Autodesk Fusion 360 part; units mm, degrees
(part 2 of 5)
sketch "Sketch2" plane through (0, 0, 22) normal (0, 0, 1) x (-1, 0, 0)
  line L0 (-259.9009, 59) -> (-249.9009, 59)
  line L1 (-249.9009, 59) -> (-249.9009, 53)
  line L2 (-249.9009, 53) -> (-259.9009, 53)
  line L3 (-259.9009, 53) -> (-259.9009, 59)
  arc A0 (-260.2748, 92.3293) -> (-257.2248, 89.2793) centre (-257.2248, 92.3293) ccw
  line L4 (-260.2748, 92.3293) -> (-260.2748, 97.7293)
  arc A1 (-257.2248, 100.7793) -> (-260.2748, 97.7293) centre (-257.2248, 97.7293) ccw
  line L5 (-257.2248, 100.7793) -> (-251.8248, 100.7793)
  arc A2 (-248.7748, 97.7293) -> (-251.8248, 100.7793) centre (-251.8248, 97.7293) ccw
  line L6 (-248.7748, 97.7293) -> (-248.7748, 92.3293)
  arc A3 (-251.8248, 89.2793) -> (-248.7748, 92.3293) centre (-251.8248, 92.3293) ccw
  line L7 (-251.8248, 89.2793) -> (-257.2248, 89.2793)
  line L8 (-263.1698, 97.5713) -> (-263.1698, 92.1713)
  arc A4 (-266.2198, 89.1213) -> (-263.1698, 92.1713) centre (-266.2198, 92.1713) ccw
  line L9 (-266.2198, 89.1213) -> (-271.6198, 89.1213)
  arc A5 (-274.6698, 92.1713) -> (-271.6198, 89.1213) centre (-271.6198, 92.1713) ccw
  line L10 (-274.6698, 92.1713) -> (-274.6698, 97.5713)
  arc A6 (-271.6198, 100.6213) -> (-274.6698, 97.5713) centre (-271.6198, 97.5713) ccw
  line L11 (-271.6198, 100.6213) -> (-266.2198, 100.6213)
  arc A7 (-263.1698, 97.5713) -> (-266.2198, 100.6213) centre (-266.2198, 97.5713) ccw
  circle A8 centre (-270.3911, 55.7056) radius 3
  circle A9 centre (-281.5411, 55.7956) radius 3
  line L12 (-248.7148, 86.5518) -> (-247.9448, 86.5518)
  arc A10 (-247.6948, 86.5414) -> (-247.9448, 86.5518) centre (-247.9448, 83.5518) ccw
  arc A11 (-247.4448, 86.5518) -> (-247.6948, 86.5414) centre (-247.4448, 83.5518) ccw
  line L13 (-247.4448, 86.5518) -> (-246.6748, 86.5518)
  arc A12 (-246.4248, 86.5414) -> (-246.6748, 86.5518) centre (-246.6748, 83.5518) ccw
  arc A13 (-246.1748, 86.5518) -> (-246.4248, 86.5414) centre (-246.1748, 83.5518) ccw
  line L14 (-246.1748, 86.5518) -> (-245.4048, 86.5518)
  arc A14 (-245.1548, 86.5414) -> (-245.4048, 86.5518) centre (-245.4048, 83.5518) ccw
  arc A15 (-244.9048, 86.5518) -> (-245.1548, 86.5414) centre (-244.9048, 83.5518) ccw
  line L15 (-244.9048, 86.5518) -> (-244.1348, 86.5518)
  arc A16 (-243.8848, 86.5414) -> (-244.1348, 86.5518) centre (-244.1348, 83.5518) ccw
  arc A17 (-243.6348, 86.5518) -> (-243.8848, 86.5414) centre (-243.6348, 83.5518) ccw
  line L16 (-243.6348, 86.5518) -> (-242.8648, 86.5518)
  arc A18 (-242.6148, 86.5414) -> (-242.8648, 86.5518) centre (-242.8648, 83.5518) ccw
  arc A19 (-242.3648, 86.5518) -> (-242.6148, 86.5414) centre (-242.3648, 83.5518) ccw
  line L17 (-242.3648, 86.5518) -> (-241.5148, 86.5518)
  arc A20 (-241.3048, 86.5445) -> (-241.5148, 86.5518) centre (-241.5148, 83.5518) ccw
  arc A21 (-241.0948, 86.5518) -> (-241.3048, 86.5445) centre (-241.0948, 83.5518) ccw
  line L18 (-241.0948, 86.5518) -> (-240.3248, 86.5518)
  arc A22 (-240.0748, 86.5414) -> (-240.3248, 86.5518) centre (-240.3248, 83.5518) ccw
  arc A23 (-239.8248, 86.5518) -> (-240.0748, 86.5414) centre (-239.8248, 83.5518) ccw
  line L19 (-239.8248, 86.5518) -> (-239.0548, 86.5518)
  arc A24 (-238.8048, 86.5414) -> (-239.0548, 86.5518) centre (-239.0548, 83.5518) ccw
  arc A25 (-238.5548, 86.5518) -> (-238.8048, 86.5414) centre (-238.5548, 83.5518) ccw
  line L20 (-238.5548, 86.5518) -> (-237.7848, 86.5518)
  arc A26 (-237.5348, 86.5414) -> (-237.7848, 86.5518) centre (-237.7848, 83.5518) ccw
  arc A27 (-237.2848, 86.5518) -> (-237.5348, 86.5414) centre (-237.2848, 83.5518) ccw
  line L21 (-237.2848, 86.5518) -> (-236.5148, 86.5518)
  arc A28 (-236.2648, 86.5414) -> (-236.5148, 86.5518) centre (-236.5148, 83.5518) ccw
  arc A29 (-236.0148, 86.5518) -> (-236.2648, 86.5414) centre (-236.0148, 83.5518) ccw
  line L22 (-236.0148, 86.5518) -> (-235.2448, 86.5518)
  arc A30 (-234.9948, 86.5414) -> (-235.2448, 86.5518) centre (-235.2448, 83.5518) ccw
  arc A31 (-234.7448, 86.5518) -> (-234.9948, 86.5414) centre (-234.7448, 83.5518) ccw
  line L23 (-234.7448, 86.5518) -> (-233.9748, 86.5518)
  arc A32 (-233.7248, 86.5414) -> (-233.9748, 86.5518) centre (-233.9748, 83.5518) ccw
  arc A33 (-233.4748, 86.5518) -> (-233.7248, 86.5414) centre (-233.4748, 83.5518) ccw
  line L24 (-233.4748, 86.5518) -> (-232.7048, 86.5518)
  arc A34 (-232.4548, 86.5414) -> (-232.7048, 86.5518) centre (-232.7048, 83.5518) ccw
  arc A35 (-232.2048, 86.5518) -> (-232.4548, 86.5414) centre (-232.2048, 83.5518) ccw
  line L25 (-232.2048, 86.5518) -> (-199.377, 86.5518)
  line L26 (-199.377, 86.5518) -> (-199.377, 118.6521)
  line L27 (-199.377, 118.6521) -> (-338.527, 118.6521)
  line L28 (-338.527, 118.6521) -> (-338.527, 36.7921)
  line L29 (-338.527, 36.7921) -> (-199.377, 36.7921)
  line L30 (-199.377, 36.7921) -> (-199.377, 62.5518)
  line L31 (-199.377, 62.5518) -> (-232.2048, 62.5518)
  arc A36 (-232.4548, 62.5622) -> (-232.2048, 62.5518) centre (-232.2048, 65.5518) ccw
  arc A37 (-232.7048, 62.5518) -> (-232.4548, 62.5622) centre (-232.7048, 65.5518) ccw
  line L32 (-232.7048, 62.5518) -> (-233.4748, 62.5518)
  arc A38 (-233.633, 62.556) -> (-233.4748, 62.5518) centre (-233.4748, 65.5518) ccw
  line L33 (-233.633, 62.556) -> (-233.633, 53)
  line L34 (-233.633, 53) -> (-245.633, 53)
  line L35 (-245.633, 53) -> (-245.633, 62.5518)
  line L36 (-245.633, 62.5518) -> (-246.1748, 62.5518)
  arc A39 (-246.4248, 62.5622) -> (-246.1748, 62.5518) centre (-246.1748, 65.5518) ccw
  arc A40 (-246.6748, 62.5518) -> (-246.4248, 62.5622) centre (-246.6748, 65.5518) ccw
  line L37 (-246.6748, 62.5518) -> (-247.4448, 62.5518)
  arc A41 (-247.6948, 62.5622) -> (-247.4448, 62.5518) centre (-247.4448, 65.5518) ccw
  arc A42 (-247.9448, 62.5518) -> (-247.6948, 62.5622) centre (-247.9448, 65.5518) ccw
  line L38 (-247.9448, 62.5518) -> (-248.7148, 62.5518)
  arc A43 (-248.9648, 62.5622) -> (-248.7148, 62.5518) centre (-248.7148, 65.5518) ccw
  arc A44 (-249.2148, 62.5518) -> (-248.9648, 62.5622) centre (-249.2148, 65.5518) ccw
  line L39 (-249.2148, 62.5518) -> (-252.4198, 62.5518)
  arc A45 (-253.4198, 63.5518) -> (-252.4198, 62.5518) centre (-252.4198, 63.5518) ccw
  line L40 (-253.4198, 63.5518) -> (-253.4198, 68.5418)
  arc A46 (-253.4094, 68.7918) -> (-253.4198, 68.5418) centre (-250.4198, 68.5418) ccw
  arc A47 (-253.4198, 69.0418) -> (-253.4094, 68.7918) centre (-250.4198, 69.0418) ccw
  line L41 (-253.4198, 69.0418) -> (-253.4198, 69.8118)
  arc A48 (-253.4094, 70.0618) -> (-253.4198, 69.8118) centre (-250.4198, 69.8118) ccw
  arc A49 (-253.4198, 70.3118) -> (-253.4094, 70.0618) centre (-250.4198, 70.3118) ccw
  line L42 (-253.4198, 70.3118) -> (-253.4198, 71.0818)
  arc A50 (-253.4094, 71.3318) -> (-253.4198, 71.0818) centre (-250.4198, 71.0818) ccw
  arc A51 (-253.4198, 71.5818) -> (-253.4094, 71.3318) centre (-250.4198, 71.5818) ccw
  line L43 (-253.4198, 71.5818) -> (-253.4198, 72.3518)
  arc A52 (-253.4094, 72.6018) -> (-253.4198, 72.3518) centre (-250.4198, 72.3518) ccw
  arc A53 (-253.4198, 72.8518) -> (-253.4094, 72.6018) centre (-250.4198, 72.8518) ccw
  line L44 (-253.4198, 72.8518) -> (-253.4198, 73.6218)
  arc A54 (-253.4094, 73.8718) -> (-253.4198, 73.6218) centre (-250.4198, 73.6218) ccw
  arc A55 (-253.4198, 74.1218) -> (-253.4094, 73.8718) centre (-250.4198, 74.1218) ccw
  line L45 (-253.4198, 74.1218) -> (-253.4198, 74.8918)
  arc A56 (-253.4094, 75.1418) -> (-253.4198, 74.8918) centre (-250.4198, 74.8918) ccw
  arc A57 (-253.4198, 75.3918) -> (-253.4094, 75.1418) centre (-250.4198, 75.3918) ccw
  line L46 (-253.4198, 75.3918) -> (-253.4198, 76.1618)
  arc A58 (-253.4094, 76.4118) -> (-253.4198, 76.1618) centre (-250.4198, 76.1618) ccw
  arc A59 (-253.4198, 76.6618) -> (-253.4094, 76.4118) centre (-250.4198, 76.6618) ccw
  line L47 (-253.4198, 76.6618) -> (-253.4198, 77.4318)
  arc A60 (-253.4094, 77.6818) -> (-253.4198, 77.4318) centre (-250.4198, 77.4318) ccw
  arc A61 (-253.4198, 77.9318) -> (-253.4094, 77.6818) centre (-250.4198, 77.9318) ccw
  line L48 (-253.4198, 77.9318) -> (-253.4198, 78.7018)
  arc A62 (-253.4094, 78.9518) -> (-253.4198, 78.7018) centre (-250.4198, 78.7018) ccw
  arc A63 (-253.4198, 79.2018) -> (-253.4094, 78.9518) centre (-250.4198, 79.2018) ccw
  line L49 (-253.4198, 79.2018) -> (-253.4198, 79.9718)
  arc A64 (-253.4094, 80.2218) -> (-253.4198, 79.9718) centre (-250.4198, 79.9718) ccw
  arc A65 (-253.4198, 80.4718) -> (-253.4094, 80.2218) centre (-250.4198, 80.4718) ccw
  line L50 (-253.4198, 80.4718) -> (-253.4198, 85.5518)
  arc A66 (-252.4198, 86.5518) -> (-253.4198, 85.5518) centre (-252.4198, 85.5518) ccw
  line L51 (-252.4198, 86.5518) -> (-249.2148, 86.5518)
  arc A67 (-248.9648, 86.5414) -> (-249.2148, 86.5518) centre (-249.2148, 83.5518) ccw
  arc A68 (-248.7148, 86.5518) -> (-248.9648, 86.5414) centre (-248.7148, 83.5518) ccw
  line L52 (-266.6857, 52.6914) -> (-273.6857, 52.6914) construction
  line L53 (-273.6857, 52.6914) -> (-273.6857, 49.6914) construction
  line L54 (-273.6857, 49.6914) -> (-266.6857, 49.6914) construction
  line L55 (-266.6857, 49.6914) -> (-266.6857, 52.6914) construction
  line L56 (-266.6857, 52.6914) -> (-273.6857, 52.6914) construction
  line L57 (-273.6857, 52.6914) -> (-273.6857, 49.6914) construction
  line L58 (-273.6857, 49.6914) -> (-266.6857, 49.6914) construction
  line L59 (-266.6857, 49.6914) -> (-266.6857, 52.6914) construction
  line L60 (-277.8686, 52.3387) -> (-283.3242, 52.3387) construction
  line L61 (-283.3242, 52.3387) -> (-283.3242, 49.9371) construction
  line L62 (-283.3242, 49.9371) -> (-277.8686, 49.9371) construction
  line L63 (-277.8686, 49.9371) -> (-277.8686, 52.3387) construction
  line L64 (-251.7291, 106.4343) -> (-265.6571, 106.4343) construction
  line L65 (-265.6571, 106.4343) -> (-265.6571, 101.6182) construction
  line L66 (-265.6571, 101.6182) -> (-251.7291, 101.6182) construction
  line L67 (-251.7291, 101.6182) -> (-251.7291, 106.4343) construction
  line L68 (-265.6571, 106.1257) -> (-277.7028, 106.1257) construction
  line L69 (-277.7028, 106.1257) -> (-277.7028, 101.6182) construction
  line L70 (-277.7028, 101.6182) -> (-265.6571, 101.6182) construction
  line L71 (-265.6571, 101.6182) -> (-265.6571, 106.1257) construction
  dimension "d91" = 2
  dimension "d93" = 2
  dimension "d95" = 2
  dimension "d97" = 2
  dimension "d99" = 2
  text T0 "Status" font "Arial" height 2 align left top in box 7 x 3 at (-266.6857, 52.6914) x (-1, 0) y (0, -1) spacing 1
  text T1 "Power" font "Arial" height 2 align left top in box 5.4557 x 2.4015 at (-277.8686, 52.3387) x (-1, 0) y (0, -1) spacing 1
  text T2 "Boot" font "Arial" height 2 align left top in box 13.928 x 4.8161 at (-251.7291, 106.4343) x (-1, 0) y (0, -1) spacing 1
  text T3 "Reset" font "Arial" height 2 align left top in box 12.0457 x 4.5075 at (-265.6571, 106.1257) x (-1, 0) y (0, -1) spacing 1
extrude "Extrude2" cut sketch "Sketch2" against normal blind 0.5 text T0 T1 T2 T3
sketch "Sketch3" plane through (0, 0, 22) normal (0, 0, 1) x (-1, 0, 0)
  line L0 (-248.7148, 86.5518) -> (-247.9448, 86.5518)
  arc A0 (-247.6948, 86.5414) -> (-247.9448, 86.5518) centre (-247.9448, 83.5518) ccw
  arc A1 (-247.4448, 86.5518) -> (-247.6948, 86.5414) centre (-247.4448, 83.5518) ccw
  line L1 (-247.4448, 86.5518) -> (-246.6748, 86.5518)
  arc A2 (-246.4248, 86.5414) -> (-246.6748, 86.5518) centre (-246.6748, 83.5518) ccw
  arc A3 (-246.1748, 86.5518) -> (-246.4248, 86.5414) centre (-246.1748, 83.5518) ccw
  line L2 (-246.1748, 86.5518) -> (-245.4048, 86.5518)
  arc A4 (-245.1548, 86.5414) -> (-245.4048, 86.5518) centre (-245.4048, 83.5518) ccw
  arc A5 (-244.9048, 86.5518) -> (-245.1548, 86.5414) centre (-244.9048, 83.5518) ccw
  line L3 (-244.9048, 86.5518) -> (-244.1348, 86.5518)
  arc A6 (-243.8848, 86.5414) -> (-244.1348, 86.5518) centre (-244.1348, 83.5518) ccw
  arc A7 (-243.6348, 86.5518) -> (-243.8848, 86.5414) centre (-243.6348, 83.5518) ccw
  line L4 (-243.6348, 86.5518) -> (-242.8648, 86.5518)
  arc A8 (-242.6148, 86.5414) -> (-242.8648, 86.5518) centre (-242.8648, 83.5518) ccw
  arc A9 (-242.3648, 86.5518) -> (-242.6148, 86.5414) centre (-242.3648, 83.5518) ccw
  line L5 (-242.3648, 86.5518) -> (-241.5148, 86.5518)
  arc A10 (-241.3048, 86.5445) -> (-241.5148, 86.5518) centre (-241.5148, 83.5518) ccw
  arc A11 (-241.0948, 86.5518) -> (-241.3048, 86.5445) centre (-241.0948, 83.5518) ccw
  line L6 (-241.0948, 86.5518) -> (-240.3248, 86.5518)
  arc A12 (-240.0748, 86.5414) -> (-240.3248, 86.5518) centre (-240.3248, 83.5518) ccw
  arc A13 (-239.8248, 86.5518) -> (-240.0748, 86.5414) centre (-239.8248, 83.5518) ccw
  line L7 (-239.8248, 86.5518) -> (-239.0548, 86.5518)
  arc A14 (-238.8048, 86.5414) -> (-239.0548, 86.5518) centre (-239.0548, 83.5518) ccw
  arc A15 (-238.5548, 86.5518) -> (-238.8048, 86.5414) centre (-238.5548, 83.5518) ccw
  line L8 (-238.5548, 86.5518) -> (-237.7848, 86.5518)
  arc A16 (-237.5348, 86.5414) -> (-237.7848, 86.5518) centre (-237.7848, 83.5518) ccw
  arc A17 (-237.2848, 86.5518) -> (-237.5348, 86.5414) centre (-237.2848, 83.5518) ccw
  line L9 (-237.2848, 86.5518) -> (-236.5148, 86.5518)
  arc A18 (-236.2648, 86.5414) -> (-236.5148, 86.5518) centre (-236.5148, 83.5518) ccw
  arc A19 (-236.0148, 86.5518) -> (-236.2648, 86.5414) centre (-236.0148, 83.5518) ccw
  line L10 (-236.0148, 86.5518) -> (-235.2448, 86.5518)
  arc A20 (-234.9948, 86.5414) -> (-235.2448, 86.5518) centre (-235.2448, 83.5518) ccw
  arc A21 (-234.7448, 86.5518) -> (-234.9948, 86.5414) centre (-234.7448, 83.5518) ccw
  line L11 (-234.7448, 86.5518) -> (-233.9748, 86.5518)
  arc A22 (-233.7248, 86.5414) -> (-233.9748, 86.5518) centre (-233.9748, 83.5518) ccw
  arc A23 (-233.4748, 86.5518) -> (-233.7248, 86.5414) centre (-233.4748, 83.5518) ccw
  line L12 (-233.4748, 86.5518) -> (-232.7048, 86.5518)
  arc A24 (-232.4548, 86.5414) -> (-232.7048, 86.5518) centre (-232.7048, 83.5518) ccw
  arc A25 (-232.2048, 86.5518) -> (-232.4548, 86.5414) centre (-232.2048, 83.5518) ccw
  line L13 (-232.2048, 86.5518) -> (-199.377, 86.5518)
  line L14 (-199.377, 86.5518) -> (-199.377, 118.6521)
  line L15 (-199.377, 118.6521) -> (-338.527, 118.6521)
  line L16 (-338.527, 118.6521) -> (-338.527, 36.7921)
  line L17 (-338.527, 36.7921) -> (-199.377, 36.7921)
  line L18 (-199.377, 36.7921) -> (-199.377, 62.5518)
  line L19 (-199.377, 62.5518) -> (-232.2048, 62.5518)
  arc A26 (-232.4548, 62.5622) -> (-232.2048, 62.5518) centre (-232.2048, 65.5518) ccw
  arc A27 (-232.7048, 62.5518) -> (-232.4548, 62.5622) centre (-232.7048, 65.5518) ccw
  line L20 (-232.7048, 62.5518) -> (-233.4748, 62.5518)
  arc A28 (-233.633, 62.556) -> (-233.4748, 62.5518) centre (-233.4748, 65.5518) ccw
  line L21 (-233.633, 62.556) -> (-233.633, 53)
  line L22 (-233.633, 53) -> (-245.633, 53)
  line L23 (-245.633, 53) -> (-245.633, 62.5518)
  line L24 (-245.633, 62.5518) -> (-246.1748, 62.5518)
  arc A29 (-246.4248, 62.5622) -> (-246.1748, 62.5518) centre (-246.1748, 65.5518) ccw
  arc A30 (-246.6748, 62.5518) -> (-246.4248, 62.5622) centre (-246.6748, 65.5518) ccw
  line L25 (-246.6748, 62.5518) -> (-247.4448, 62.5518)
  arc A31 (-247.6948, 62.5622) -> (-247.4448, 62.5518) centre (-247.4448, 65.5518) ccw
  arc A32 (-247.9448, 62.5518) -> (-247.6948, 62.5622) centre (-247.9448, 65.5518) ccw
  line L26 (-247.9448, 62.5518) -> (-248.7148, 62.5518)
  arc A33 (-248.9648, 62.5622) -> (-248.7148, 62.5518) centre (-248.7148, 65.5518) ccw
  arc A34 (-249.2148, 62.5518) -> (-248.9648, 62.5622) centre (-249.2148, 65.5518) ccw
  line L27 (-249.2148, 62.5518) -> (-252.4198, 62.5518)
  arc A35 (-253.4198, 63.5518) -> (-252.4198, 62.5518) centre (-252.4198, 63.5518) ccw
  line L28 (-253.4198, 63.5518) -> (-253.4198, 68.5418)
  arc A36 (-253.4094, 68.7918) -> (-253.4198, 68.5418) centre (-250.4198, 68.5418) ccw
  arc A37 (-253.4198, 69.0418) -> (-253.4094, 68.7918) centre (-250.4198, 69.0418) ccw
  line L29 (-253.4198, 69.0418) -> (-253.4198, 69.8118)
  arc A38 (-253.4094, 70.0618) -> (-253.4198, 69.8118) centre (-250.4198, 69.8118) ccw
  arc A39 (-253.4198, 70.3118) -> (-253.4094, 70.0618) centre (-250.4198, 70.3118) ccw
  line L30 (-253.4198, 70.3118) -> (-253.4198, 71.0818)
  arc A40 (-253.4094, 71.3318) -> (-253.4198, 71.0818) centre (-250.4198, 71.0818) ccw
  arc A41 (-253.4198, 71.5818) -> (-253.4094, 71.3318) centre (-250.4198, 71.5818) ccw
  line L31 (-253.4198, 71.5818) -> (-253.4198, 72.3518)
  arc A42 (-253.4094, 72.6018) -> (-253.4198, 72.3518) centre (-250.4198, 72.3518) ccw
  arc A43 (-253.4198, 72.8518) -> (-253.4094, 72.6018) centre (-250.4198, 72.8518) ccw
  line L32 (-253.4198, 72.8518) -> (-253.4198, 73.6218)
  arc A44 (-253.4094, 73.8718) -> (-253.4198, 73.6218) centre (-250.4198, 73.6218) ccw
  arc A45 (-253.4198, 74.1218) -> (-253.4094, 73.8718) centre (-250.4198, 74.1218) ccw
  line L33 (-253.4198, 74.1218) -> (-253.4198, 74.8918)
  arc A46 (-253.4094, 75.1418) -> (-253.4198, 74.8918) centre (-250.4198, 74.8918) ccw
  arc A47 (-253.4198, 75.3918) -> (-253.4094, 75.1418) centre (-250.4198, 75.3918) ccw
  line L34 (-253.4198, 75.3918) -> (-253.4198, 76.1618)
  arc A48 (-253.4094, 76.4118) -> (-253.4198, 76.1618) centre (-250.4198, 76.1618) ccw
  arc A49 (-253.4198, 76.6618) -> (-253.4094, 76.4118) centre (-250.4198, 76.6618) ccw
  line L35 (-253.4198, 76.6618) -> (-253.4198, 77.4318)
  arc A50 (-253.4094, 77.6818) -> (-253.4198, 77.4318) centre (-250.4198, 77.4318) ccw
  arc A51 (-253.4198, 77.9318) -> (-253.4094, 77.6818) centre (-250.4198, 77.9318) ccw
  line L36 (-253.4198, 77.9318) -> (-253.4198, 78.7018)
  arc A52 (-253.4094, 78.9518) -> (-253.4198, 78.7018) centre (-250.4198, 78.7018) ccw
  arc A53 (-253.4198, 79.2018) -> (-253.4094, 78.9518) centre (-250.4198, 79.2018) ccw
  line L37 (-253.4198, 79.2018) -> (-253.4198, 79.9718)
  arc A54 (-253.4094, 80.2218) -> (-253.4198, 79.9718) centre (-250.4198, 79.9718) ccw
  arc A55 (-253.4198, 80.4718) -> (-253.4094, 80.2218) centre (-250.4198, 80.4718) ccw
  line L38 (-253.4198, 80.4718) -> (-253.4198, 85.5518)
  arc A56 (-252.4198, 86.5518) -> (-253.4198, 85.5518) centre (-252.4198, 85.5518) ccw
  line L39 (-252.4198, 86.5518) -> (-249.2148, 86.5518)
  arc A57 (-248.9648, 86.5414) -> (-249.2148, 86.5518) centre (-249.2148, 83.5518) ccw
  arc A58 (-248.7148, 86.5518) -> (-248.9648, 86.5414) centre (-248.7148, 83.5518) ccw
  circle A59 centre (-281.5411, 55.7956) radius 3
  circle A60 centre (-270.3911, 55.7056) radius 3
  line L40 (-263.1698, 97.5713) -> (-263.1698, 92.1713)
  arc A61 (-266.2198, 89.1213) -> (-263.1698, 92.1713) centre (-266.2198, 92.1713) ccw
  line L41 (-266.2198, 89.1213) -> (-271.6198, 89.1213)
  arc A62 (-274.6698, 92.1713) -> (-271.6198, 89.1213) centre (-271.6198, 92.1713) ccw
  line L42 (-274.6698, 92.1713) -> (-274.6698, 97.5713)
  arc A63 (-271.6198, 100.6213) -> (-274.6698, 97.5713) centre (-271.6198, 97.5713) ccw
  line L43 (-271.6198, 100.6213) -> (-266.2198, 100.6213)
  arc A64 (-263.1698, 97.5713) -> (-266.2198, 100.6213) centre (-266.2198, 97.5713) ccw
  arc A65 (-260.2748, 92.3293) -> (-257.2248, 89.2793) centre (-257.2248, 92.3293) ccw
  line L44 (-260.2748, 92.3293) -> (-260.2748, 97.7293)
  arc A66 (-257.2248, 100.7793) -> (-260.2748, 97.7293) centre (-257.2248, 97.7293) ccw
  line L45 (-257.2248, 100.7793) -> (-251.8248, 100.7793)
  arc A67 (-248.7748, 97.7293) -> (-251.8248, 100.7793) centre (-251.8248, 97.7293) ccw
  line L46 (-248.7748, 97.7293) -> (-248.7748, 92.3293)
  arc A68 (-251.8248, 89.2793) -> (-248.7748, 92.3293) centre (-251.8248, 92.3293) ccw
  line L47 (-251.8248, 89.2793) -> (-257.2248, 89.2793)
  line L48 (-259.9009, 59) -> (-249.9009, 59)
  line L49 (-249.9009, 59) -> (-249.9009, 53)
  line L50 (-249.9009, 53) -> (-259.9009, 53)
  line L51 (-259.9009, 53) -> (-259.9009, 59)
  line L52 (-265.9218, 103.6182) -> (-265.6571, 103.6182)
  line L53 (-265.6571, 103.6182) -> (-265.6571, 101.6182)
  spline S0 degree 3 poles (-266.9504, 101.6721) (-266.9947, 101.6939) (-267.085, 101.7384) (-267.1432, 101.8206) (-267.1728, 101.8624) knots 0 0 0 0 0.014568 0.029686 0.029686 0.029686 0.029686
  spline S1 degree 3 poles (-267.1728, 101.8624) (-267.1971, 101.9093) (-267.246, 102.004) (-267.2527, 102.1103) (-267.256, 102.1639) knots 0 0 0 0 0.015657 0.031584 0.031584 0.031584 0.031584
  spline S2 degree 3 poles (-272.5725, 103.4081) (-272.5883, 103.4076) (-272.6244, 103.4063) (-272.6602, 103.4014) (-272.6803, 103.3986) knots 0 0 0 0 0.004747 0.010826 0.010826 0.010826 0.010826
  line L54 (-272.6803, 103.3986) -> (-272.7158, 103.6155)
  spline S3 degree 3 poles (-271.4306, 103.3781) (-271.4615, 103.349) (-271.529, 103.2853) (-271.5634, 103.1987) (-271.5821, 103.1517) knots 0 0 0 0 0.012573 0.027537 0.027537 0.027537 0.027537
  line L55 (-271.5821, 103.1517) -> (-271.8358, 103.183)
  spline S4 degree 3 poles (-271.8358, 103.183) (-271.8125, 103.2523) (-271.7674, 103.3862) (-271.6636, 103.4819) (-271.6134, 103.5282) knots 0 0 0 0 0.021523 0.041652 0.041652 0.041652 0.041652
  spline S5 degree 3 poles (-254.1602, 103.651) (-254.0648, 103.644) (-253.88, 103.6304) (-253.7373, 103.5128) (-253.6684, 103.4559) knots 0 0 0 0 0.027936 0.054087 0.054087 0.054087 0.054087
  spline S6 degree 3 poles (-253.6684, 103.4559) (-253.6138, 103.3793) (-253.4945, 103.2119) (-253.4856, 103.0056) (-253.4808, 102.8938) knots 0 0 0 0 0.027653 0.060391 0.060391 0.060391 0.060391
  spline S7 degree 3 poles (-253.4808, 102.8938) (-253.4864, 102.7719) (-253.4967, 102.5476) (-253.6394, 102.3759) (-253.7045, 102.2976) knots 0 0 0 0 0.035471 0.065242 0.065242 0.065242 0.065242
  spline S8 degree 3 poles (-253.7045, 102.2976) (-253.7713, 102.2507) (-253.9079, 102.1545) (-254.0748, 102.1427) (-254.1602, 102.1367) knots 0 0 0 0 0.023996 0.049149 0.049149 0.049149 0.049149
  spline S9 degree 3 poles (-254.1602, 102.1367) (-254.2544, 102.1439) (-254.438, 102.1581) (-254.5796, 102.2753) (-254.6486, 102.3324) knots 0 0 0 0 0.027586 0.05378 0.05378 0.05378 0.05378
  spline S10 degree 3 poles (-254.6486, 102.3324) (-254.7038, 102.4073) (-254.8221, 102.5675) (-254.8326, 102.767) (-254.8382, 102.8734) knots 0 0 0 0 0.027308 0.058452 0.058452 0.058452 0.058452
  spline S11 degree 3 poles (-254.8382, 102.8734) (-254.8366, 102.9577) (-254.8336, 103.1095) (-254.7787, 103.2506) (-254.7543, 103.3133) knots 0 0 0 0 0.025071 0.045099 0.045099 0.045099 0.045099
  spline S12 degree 3 poles (-254.7543, 103.3133) (-254.7231, 103.3638) (-254.6604, 103.4652) (-254.5603, 103.5298) (-254.5101, 103.5623) knots 0 0 0 0 0.017574 0.035265 0.035265 0.035265 0.035265
  spline S13 degree 3 poles (-254.5101, 103.5623) (-254.4552, 103.5882) (-254.3443, 103.6404) (-254.2219, 103.6474) (-254.1602, 103.651) knots 0 0 0 0 0.018034 0.036399 0.036399 0.036399 0.036399
  spline S14 degree 3 poles (-255.7141, 103.651) (-255.6186, 103.644) (-255.4339, 103.6304) (-255.2912, 103.5128) (-255.2223, 103.4559) knots 0 0 0 0 0.027936 0.054087 0.054087 0.054087 0.054087
  spline S15 degree 3 poles (-255.2223, 103.4559) (-255.1677, 103.3793) (-255.0484, 103.2119) (-255.0395, 103.0056) (-255.0347, 102.8938) knots 0 0 0 0 0.027653 0.060391 0.060391 0.060391 0.060391
  spline S16 degree 3 poles (-255.0347, 102.8938) (-255.0403, 102.7719) (-255.0506, 102.5476) (-255.1933, 102.3759) (-255.2584, 102.2976) knots 0 0 0 0 0.035471 0.065242 0.065242 0.065242 0.065242
  spline S17 degree 3 poles (-255.2584, 102.2976) (-255.3251, 102.2507) (-255.4618, 102.1545) (-255.6287, 102.1427) (-255.7141, 102.1367) knots 0 0 0 0 0.023996 0.049149 0.049149 0.049149 0.049149
  spline S18 degree 3 poles (-255.7141, 102.1367) (-255.8083, 102.1439) (-255.9918, 102.1581) (-256.1335, 102.2753) (-256.2025, 102.3324) knots 0 0 0 0 0.027586 0.05378 0.05378 0.05378 0.05378
  spline S19 degree 3 poles (-256.2025, 102.3324) (-256.2577, 102.4073) (-256.376, 102.5675) (-256.3865, 102.767) (-256.3921, 102.8734) knots 0 0 0 0 0.027308 0.058452 0.058452 0.058452 0.058452
  spline S20 degree 3 poles (-256.3921, 102.8734) (-256.3905, 102.9577) (-256.3875, 103.1095) (-256.3326, 103.2506) (-256.3082, 103.3133) knots 0 0 0 0 0.025071 0.045099 0.045099 0.045099 0.045099
  spline S21 degree 3 poles (-256.3082, 103.3133) (-256.277, 103.3638) (-256.2143, 103.4652) (-256.1142, 103.5298) (-256.064, 103.5623) knots 0 0 0 0 0.017574 0.035265 0.035265 0.035265 0.035265
  spline S22 degree 3 poles (-256.064, 103.5623) (-256.0091, 103.5882) (-255.8982, 103.6404) (-255.7758, 103.6474) (-255.7141, 103.651) knots 0 0 0 0 0.018034 0.036399 0.036399 0.036399 0.036399
  spline S23 degree 3 poles (-280.2888, 51.9699) (-280.1933, 51.9629) (-280.0086, 51.9493) (-279.8659, 51.8317) (-279.797, 51.7748) knots 0 0 0 0 0.027936 0.054087 0.054087 0.054087 0.054087
  spline S24 degree 3 poles (-279.797, 51.7748) (-279.7424, 51.6982) (-279.6231, 51.5308) (-279.6142, 51.3245) (-279.6094, 51.2127) knots 0 0 0 0 0.027653 0.060391 0.060391 0.060391 0.060391
  spline S25 degree 3 poles (-279.6094, 51.2127) (-279.615, 51.0908) (-279.6253, 50.8665) (-279.768, 50.6949) (-279.8331, 50.6165) knots 0 0 0 0 0.035471 0.065242 0.065242 0.065242 0.065242
  spline S26 degree 3 poles (-279.8331, 50.6165) (-279.8998, 50.5696) (-280.0365, 50.4734) (-280.2034, 50.4616) (-280.2888, 50.4556) knots 0 0 0 0 0.023996 0.049149 0.049149 0.049149 0.049149
  spline S27 degree 3 poles (-280.2888, 50.4556) (-280.383, 50.4628) (-280.5665, 50.477) (-280.7082, 50.5942) (-280.7772, 50.6513) knots 0 0 0 0 0.027586 0.05378 0.05378 0.05378 0.05378
  spline S28 degree 3 poles (-280.7772, 50.6513) (-280.8324, 50.7262) (-280.9507, 50.8864) (-280.9612, 51.0859) (-280.9668, 51.1923) knots 0 0 0 0 0.027308 0.058452 0.058452 0.058452 0.058452
  spline S29 degree 3 poles (-280.9668, 51.1923) (-280.9652, 51.2766) (-280.9622, 51.4284) (-280.9073, 51.5696) (-280.8829, 51.6322) knots 0 0 0 0 0.025071 0.045099 0.045099 0.045099 0.045099
  spline S30 degree 3 poles (-280.8829, 51.6322) (-280.8517, 51.6827) (-280.789, 51.7841) (-280.6889, 51.8488) (-280.6387, 51.8812) knots 0 0 0 0 0.017574 0.035265 0.035265 0.035265 0.035265
  spline S31 degree 3 poles (-280.6387, 51.8812) (-280.5838, 51.9071) (-280.4729, 51.9593) (-280.3505, 51.9663) (-280.2888, 51.9699) knots 0 0 0 0 0.018034 0.036399 0.036399 0.036399 0.036399
  line L56 (-282.0719, 50.8225) -> (-281.7785, 51.9371)
  line L57 (-281.7785, 51.9371) -> (-281.5221, 51.9371)
  line L58 (-281.5221, 51.9371) -> (-281.0787, 50.4883)
  line L59 (-281.0787, 50.4883) -> (-281.3324, 50.4883)
  line L60 (-281.3324, 50.4883) -> (-281.563, 51.3246)
  line L61 (-281.563, 51.3246) -> (-281.6489, 51.6356)
  spline S32 degree 3 poles (-281.6489, 51.6356) (-281.6561, 51.6069) (-281.6809, 51.5072) (-281.7061, 51.4077) (-281.724, 51.3369) knots 0 0 0 0 0.008892 0.030805 0.030805 0.030805 0.030805
  line L62 (-281.724, 51.3369) -> (-281.9545, 50.4883)
  line L63 (-281.9545, 50.4883) -> (-282.2069, 50.4883)
  line L64 (-282.2069, 50.4883) -> (-282.4238, 51.3287)
  line L65 (-282.4238, 51.3287) -> (-282.4961, 51.6056)
  line L66 (-282.4961, 51.6056) -> (-282.5794, 51.326)
  line L67 (-282.5794, 51.326) -> (-282.8277, 50.4883)
  line L68 (-282.8277, 50.4883) -> (-283.0664, 50.4883)
  line L69 (-283.0664, 50.4883) -> (-282.6135, 51.9371)
  line L70 (-282.6135, 51.9371) -> (-282.3584, 51.9371)
  line L71 (-282.3584, 51.9371) -> (-282.1278, 51.0695)
  line L72 (-282.1278, 51.0695) -> (-282.0719, 50.8225)
  spline S33 degree 3 poles (-266.5439, 101.6182) (-266.6229, 101.6188) (-266.7608, 101.6199) (-266.8937, 101.6565) (-266.9504, 101.6721) knots 0 0 0 0 0.023572 0.041164 0.041164 0.041164 0.041164
  spline S34 degree 3 poles (-266.7955, 51.4083) (-266.7649, 51.3532) (-266.7026, 51.2412) (-266.6914, 51.1136) (-266.6857, 51.0489) knots 0 0 0 0 0.018713 0.037965 0.037965 0.037965 0.037965
  line L73 (-266.6857, 51.0489) -> (-266.9354, 51.027)
  spline S35 degree 3 poles (-266.9354, 51.027) (-266.9424, 51.0735) (-266.9556, 51.1605) (-266.9981, 51.2375) (-267.0179, 51.2733) knots 0 0 0 0 0.013975 0.026155 0.026155 0.026155 0.026155
  spline S36 degree 3 poles (-267.0179, 51.2733) (-267.0438, 51.3044) (-267.0993, 51.3709) (-267.1775, 51.4087) (-267.2191, 51.4288) knots 0 0 0 0 0.012002 0.025694 0.025694 0.025694 0.025694
  spline S37 degree 3 poles (-267.2191, 51.4288) (-267.267, 51.4461) (-267.3661, 51.482) (-267.4715, 51.486) (-267.5261, 51.4881) knots 0 0 0 0 0.015163 0.031432 0.031432 0.031432 0.031432
  spline S38 degree 3 poles (-267.5261, 51.4881) (-267.574, 51.4867) (-267.6653, 51.4839) (-267.7522, 51.4563) (-267.7935, 51.4431) knots 0 0 0 0 0.014301 0.027232 0.027232 0.027232 0.027232
  spline S39 degree 3 poles (-267.7935, 51.4431) (-267.8289, 51.4277) (-267.8954, 51.3988) (-267.9436, 51.3448) (-267.9661, 51.3197) knots 0 0 0 0 0.011435 0.021444 0.021444 0.021444 0.021444
  spline S40 degree 3 poles (-267.9661, 51.3197) (-267.9826, 51.2931) (-268.0152, 51.2406) (-268.0202, 51.1789) (-268.0227, 51.1484) knots 0 0 0 0 0.009237 0.018267 0.018267 0.018267 0.018267
  spline S41 degree 3 poles (-268.0227, 51.1484) (-268.0206, 51.1183) (-268.0164, 51.0588) (-267.984, 51.0087) (-267.9681, 50.9841) knots 0 0 0 0 0.008921 0.017573 0.017573 0.017573 0.017573
  spline S42 degree 3 poles (-267.9681, 50.9841) (-267.9451, 50.9609) (-267.8935, 50.909) (-267.8256, 50.8814) (-267.788, 50.866) knots 0 0 0 0 0.009698 0.021725 0.021725 0.021725 0.021725
  spline S43 degree 3 poles (-267.788, 50.866) (-267.7451, 50.8523) (-267.6278, 50.8147) (-267.5079, 50.7864) (-267.432, 50.7685) knots 0 0 0 0 0.013533 0.036931 0.036931 0.036931 0.036931
  spline S44 degree 3 poles (-267.432, 50.7685) (-267.353, 50.7496) (-267.2209, 50.7181) (-267.0961, 50.665) (-267.0459, 50.6437) knots 0 0 0 0 0.024297 0.040637 0.040637 0.040637 0.040637
  spline S45 degree 3 poles (-267.0459, 50.6437) (-267.0019, 50.6183) (-266.9185, 50.5701) (-266.86, 50.4936) (-266.8324, 50.4575) knots 0 0 0 0 0.015064 0.02858 0.02858 0.02858 0.02858
  spline S46 degree 3 poles (-266.8324, 50.4575) (-266.8119, 50.419) (-266.7704, 50.3411) (-266.7649, 50.2531) (-266.7621, 50.2085) knots 0 0 0 0 0.012908 0.026139 0.026139 0.026139 0.026139
  spline S47 degree 3 poles (-266.7621, 50.2085) (-266.7658, 50.1586) (-266.7734, 50.0579) (-266.823, 49.9698) (-266.8481, 49.9254) knots 0 0 0 0 0.014805 0.02991 0.02991 0.02991 0.02991
  spline S48 degree 3 poles (-266.8481, 49.9254) (-266.8809, 49.8838) (-266.9489, 49.7977) (-267.0479, 49.7501) (-267.0991, 49.7255) knots 0 0 0 0 0.01568 0.032466 0.032466 0.032466 0.032466
  spline S49 degree 3 poles (-267.0991, 49.7255) (-267.1566, 49.7056) (-267.2755, 49.6646) (-267.4012, 49.6598) (-267.4661, 49.6573) knots 0 0 0 0 0.018164 0.037509 0.037509 0.037509 0.037509
  spline S50 degree 3 poles (-267.4661, 49.6573) (-267.5365, 49.6597) (-267.6709, 49.6642) (-267.7979, 49.7081) (-267.8583, 49.7289) knots 0 0 0 0 0.021001 0.040071 0.040071 0.040071 0.040071
  spline S51 degree 3 poles (-267.8583, 49.7289) (-267.9112, 49.755) (-268.0142, 49.8056) (-268.0851, 49.8958) (-268.1196, 49.9397) knots 0 0 0 0 0.017437 0.033952 0.033952 0.033952 0.033952
  spline S52 degree 3 poles (-268.1196, 49.9397) (-268.1465, 49.9881) (-268.2012, 50.0862) (-268.2122, 50.1981) (-268.2178, 50.2549) knots 0 0 0 0 0.016416 0.033327 0.033327 0.033327 0.033327
  line L74 (-268.2178, 50.2549) -> (-267.964, 50.274)
  spline S53 degree 3 poles (-267.964, 50.274) (-267.9545, 50.2158) (-267.9365, 50.1062) (-267.861, 50.0254) (-267.8256, 49.9875) knots 0 0 0 0 0.017238 0.032462 0.032462 0.032462 0.032462
  spline S54 degree 3 poles (-267.8256, 49.9875) (-267.778, 49.9593) (-267.6711, 49.896) (-267.5463, 49.8925) (-267.477, 49.8906) knots 0 0 0 0 0.016321 0.036707 0.036707 0.036707 0.036707
  spline S55 degree 3 poles (-267.477, 49.8906) (-267.4061, 49.8917) (-267.2818, 49.8936) (-267.1735, 49.9531) (-267.1271, 49.9786) knots 0 0 0 0 0.02087 0.036564 0.036564 0.036564 0.036564
  spline S56 degree 3 poles (-267.1271, 49.9786) (-267.095, 50.0086) (-267.0332, 50.0666) (-267.0224, 50.1504) (-267.0172, 50.1907) knots 0 0 0 0 0.012728 0.024562 0.024562 0.024562 0.024562
  spline S57 degree 3 poles (-267.0172, 50.1907) (-267.0204, 50.225) (-267.0265, 50.2928) (-267.0723, 50.3431) (-267.095, 50.3681) knots 0 0 0 0 0.010013 0.019843 0.019843 0.019843 0.019843
  spline S58 degree 3 poles (-267.095, 50.3681) (-267.1403, 50.3933) (-267.2648, 50.4627) (-267.4049, 50.492) (-267.494, 50.5107) knots 0 0 0 0 0.01549 0.042576 0.042576 0.042576 0.042576
  spline S59 degree 3 poles (-267.494, 50.5107) (-267.5854, 50.5311) (-267.7357, 50.5646) (-267.8801, 50.6175) (-267.9367, 50.6382) knots 0 0 0 0 0.028046 0.046113 0.046113 0.046113 0.046113
  spline S60 degree 3 poles (-267.9367, 50.6382) (-267.99, 50.6653) (-268.0899, 50.716) (-268.1613, 50.802) (-268.1946, 50.8422) knots 0 0 0 0 0.017708 0.033187 0.033187 0.033187 0.033187
  spline S61 degree 3 poles (-268.1946, 50.8422) (-268.2189, 50.8854) (-268.2684, 50.9738) (-268.2746, 51.075) (-268.2778, 51.1266) knots 0 0 0 0 0.014678 0.02998 0.02998 0.02998 0.02998
  spline S62 degree 3 poles (-268.2778, 51.1266) (-268.2738, 51.1794) (-268.2656, 51.2864) (-268.2131, 51.38) (-268.1864, 51.4274) knots 0 0 0 0 0.015669 0.031781 0.031781 0.031781 0.031781
  spline S63 degree 3 poles (-268.1864, 51.4274) (-268.1518, 51.4723) (-268.0804, 51.5647) (-267.977, 51.6191) (-267.9238, 51.6471) knots 0 0 0 0 0.016779 0.034595 0.034595 0.034595 0.034595
  spline S64 degree 3 poles (-267.9238, 51.6471) (-267.8638, 51.67) (-267.7397, 51.7173) (-267.607, 51.7227) (-267.5384, 51.7255) knots 0 0 0 0 0.019123 0.039562 0.039562 0.039562 0.039562
  line L75 (-270.6352, 51.6914) -> (-270.3788, 51.6914)
  spline S65 degree 3 poles (-270.3788, 51.6914) (-270.3671, 51.6641) (-270.3426, 51.6068) (-270.3341, 51.5451) (-270.3297, 51.5127) knots 0 0 0 0 0.008862 0.018609 0.018609 0.018609 0.018609
  spline S66 degree 3 poles (-270.3297, 51.5127) (-270.2864, 51.5478) (-270.2056, 51.6134) (-270.1109, 51.6564) (-270.067, 51.6764) knots 0 0 0 0 0.016644 0.031058 0.031058 0.031058 0.031058
  spline S67 degree 3 poles (-270.067, 51.6764) (-270.0238, 51.6903) (-269.9357, 51.7187) (-269.8433, 51.7223) (-269.7962, 51.7242) knots 0 0 0 0 0.013561 0.027613 0.027613 0.027613 0.027613
  spline S68 degree 3 poles (-269.7962, 51.7242) (-269.7236, 51.7213) (-269.59, 51.7159) (-269.4796, 51.6415) (-269.4292, 51.6075) knots 0 0 0 0 0.021312 0.039186 0.039186 0.039186 0.039186
  spline S69 degree 3 poles (-269.4292, 51.6075) (-269.3918, 51.5656) (-269.3161, 51.4805) (-269.3061, 51.367) (-269.301, 51.3094) knots 0 0 0 0 0.016401 0.033233 0.033233 0.033233 0.033233
  spline S70 degree 3 poles (-269.301, 51.3094) (-269.3029, 51.275) (-269.3066, 51.207) (-269.3353, 51.1454) (-269.3494, 51.115) knots 0 0 0 0 0.010253 0.020199 0.020199 0.020199 0.020199
  spline S71 degree 3 poles (-269.3494, 51.115) (-269.3666, 51.0873) (-269.4005, 51.0326) (-269.4513, 50.9932) (-269.4763, 50.9738) knots 0 0 0 0 0.009704 0.019119 0.019119 0.019119 0.019119
  spline S72 degree 3 poles (-269.4763, 50.9738) (-269.5036, 50.9571) (-269.5591, 50.923) (-269.6213, 50.9033) (-269.653, 50.8933) knots 0 0 0 0 0.009559 0.019479 0.019479 0.019479 0.019479
  spline S73 degree 3 poles (-269.653, 50.8933) (-269.6832, 50.8867) (-269.7553, 50.8708) (-269.8286, 50.8617) (-269.8713, 50.8565) knots 0 0 0 0 0.009264 0.022147 0.022147 0.022147 0.022147
  spline S74 degree 3 poles (-269.8713, 50.8565) (-269.9578, 50.846) (-270.1059, 50.8281) (-270.2495, 50.7884) (-270.3092, 50.7719) knots 0 0 0 0 0.02611 0.044656 0.044656 0.044656 0.044656
  spline S75 degree 3 poles (-270.3092, 50.7719) (-270.3096, 50.7582) (-270.3102, 50.7368) (-270.3105, 50.7154) (-270.3106, 50.7078) knots 0 0 0 0 0.004128 0.006414 0.006414 0.006414 0.006414
  spline S76 degree 3 poles (-270.3106, 50.7078) (-270.3096, 50.6634) (-270.3078, 50.5852) (-270.2612, 50.5232) (-270.241, 50.4963) knots 0 0 0 0 0.012908 0.022759 0.022759 0.022759 0.022759
  spline S77 degree 3 poles (-270.241, 50.4963) (-270.2031, 50.4721) (-270.1183, 50.418) (-270.0172, 50.4149) (-269.9613, 50.4131) knots 0 0 0 0 0.013259 0.029661 0.029661 0.029661 0.029661
  spline S78 degree 3 poles (-269.9613, 50.4131) (-269.91, 50.4139) (-269.8198, 50.4153) (-269.7399, 50.4562) (-269.7055, 50.4738) knots 0 0 0 0 0.015134 0.026599 0.026599 0.026599 0.026599
  spline S79 degree 3 poles (-269.7055, 50.4738) (-269.6792, 50.5004) (-269.6196, 50.5608) (-269.5964, 50.6428) (-269.5834, 50.6887) knots 0 0 0 0 0.011056 0.025069 0.025069 0.025069 0.025069
  line L76 (-269.5834, 50.6887) -> (-269.3433, 50.656)
  spline S80 degree 3 poles (-269.3433, 50.656) (-269.355, 50.6083) (-269.3769, 50.5191) (-269.4275, 50.4426) (-269.4511, 50.407) knots 0 0 0 0 0.01459 0.02731 0.02731 0.02731 0.02731
  spline S81 degree 3 poles (-269.4511, 50.407) (-269.4801, 50.3768) (-269.5418, 50.3126) (-269.6243, 50.2789) (-269.668, 50.261) knots 0 0 0 0 0.012433 0.026404 0.026404 0.026404 0.026404
  spline S82 degree 3 poles (-269.668, 50.261) (-269.7187, 50.2461) (-269.826, 50.2145) (-269.9378, 50.2115) (-269.9968, 50.2098) knots 0 0 0 0 0.015787 0.033398 0.033398 0.033398 0.033398
  spline S83 degree 3 poles (-269.9968, 50.2098) (-270.0532, 50.2108) (-270.1557, 50.2125) (-270.2541, 50.2408) (-270.2983, 50.2535) knots 0 0 0 0 0.01685 0.030582 0.030582 0.030582 0.030582
  spline S84 degree 3 poles (-270.2983, 50.2535) (-270.3333, 50.2677) (-270.3971, 50.2937) (-270.4465, 50.3416) (-270.4688, 50.3633) knots 0 0 0 0 0.011204 0.020452 0.020452 0.020452 0.020452
  spline S85 degree 3 poles (-270.4688, 50.3633) (-270.4858, 50.3876) (-270.5215, 50.4385) (-270.537, 50.4988) (-270.5452, 50.5304) knots 0 0 0 0 0.008807 0.018509 0.018509 0.018509 0.018509
  spline S86 degree 3 poles (-270.5452, 50.5304) (-270.5487, 50.5597) (-270.5578, 50.6349) (-270.5576, 50.7107) (-270.5575, 50.7569) knots 0 0 0 0 0.008848 0.022698 0.022698 0.022698 0.022698
  line L77 (-270.5575, 50.7569) -> (-270.5575, 51.0843)
  spline S87 degree 3 poles (-270.5575, 51.0843) (-270.5569, 51.1776) (-270.556, 51.3222) (-270.5687, 51.4663) (-270.5732, 51.5175) knots 0 0 0 0 0.027953 0.043363 0.043363 0.043363 0.043363
  spline S88 degree 3 poles (-270.5732, 51.5175) (-270.5797, 51.5475) (-270.593, 51.6082) (-270.6211, 51.6635) (-270.6352, 51.6914) knots 0 0 0 0 0.009187 0.018535 0.018535 0.018535 0.018535
  spline S89 degree 3 poles (-271.2826, 51.4636) (-271.2943, 51.4687) (-271.3209, 51.4805) (-271.3501, 51.481) (-271.3665, 51.4813) knots 0 0 0 0 0.003804 0.008651 0.008651 0.008651 0.008651
  spline S90 degree 3 poles (-271.3665, 51.4813) (-271.3823, 51.4808) (-271.4184, 51.4795) (-271.4542, 51.4745) (-271.4743, 51.4718) knots 0 0 0 0 0.004747 0.010826 0.010826 0.010826 0.010826
  line L78 (-271.4743, 51.4718) -> (-271.5097, 51.6887)
  spline S91 degree 3 poles (-271.5097, 51.6887) (-271.4771, 51.6951) (-271.4158, 51.707) (-271.3534, 51.7094) (-271.3242, 51.7105) knots 0 0 0 0 0.009958 0.018706 0.018706 0.018706 0.018706
  spline S92 degree 3 poles (-271.3242, 51.7105) (-271.284, 51.7098) (-271.2121, 51.7084) (-271.146, 51.6805) (-271.1168, 51.6682) knots 0 0 0 0 0.011916 0.021334 0.021334 0.021334 0.021334
  spline S93 degree 3 poles (-271.1168, 51.6682) (-271.0943, 51.6534) (-271.0506, 51.6248) (-271.0253, 51.5791) (-271.0131, 51.557) knots 0 0 0 0 0.007958 0.015408 0.015408 0.015408 0.015408
  spline S94 degree 3 poles (-271.0131, 51.557) (-271.0045, 51.5215) (-270.9814, 51.4265) (-270.9825, 51.3285) (-270.9831, 51.2671) knots 0 0 0 0 0.010927 0.02924 0.02924 0.02924 0.02924
  line L79 (-270.9831, 51.2671) -> (-270.9831, 50.4336)
  line L80 (-270.9831, 50.4336) -> (-270.803, 50.4336)
  line L81 (-270.803, 50.4336) -> (-270.803, 50.2426)
  line L82 (-270.803, 50.2426) -> (-270.9831, 50.2426)
  line L83 (-270.9831, 50.2426) -> (-270.9831, 49.8838)
  line L84 (-270.9831, 49.8838) -> (-271.2273, 49.7364)
  line L85 (-271.2273, 49.7364) -> (-271.2273, 50.2426)
  line L86 (-271.2273, 50.2426) -> (-271.4743, 50.2426)
  line L87 (-271.4743, 50.2426) -> (-271.4743, 50.4336)
  line L88 (-271.4743, 50.4336) -> (-271.2273, 50.4336)
  line L89 (-271.2273, 50.4336) -> (-271.2273, 51.2808)
  spline S95 degree 3 poles (-271.2273, 51.2808) (-271.227, 51.3097) (-271.2264, 51.3553) (-271.2366, 51.3996) (-271.2403, 51.4158) knots 0 0 0 0 0.008635 0.013608 0.013608 0.013608 0.013608
  spline S96 degree 3 poles (-271.2403, 51.4158) (-271.2454, 51.4254) (-271.2556, 51.4447) (-271.2735, 51.4572) (-271.2826, 51.4636) knots 0 0 0 0 0.003189 0.00646 0.00646 0.00646 0.00646
  line L90 (-272.8835, 50.2426) -> (-272.8835, 51.6914)
  line L91 (-272.8835, 51.6914) -> (-272.6639, 51.6914)
  line L92 (-272.6639, 51.6914) -> (-272.6639, 51.4786)
  spline S97 degree 3 poles (-271.6134, 103.5282) (-271.5534, 103.564) (-271.4259, 103.6399) (-271.2773, 103.6472) (-271.1987, 103.651) knots 0 0 0 0 0.020652 0.043844 0.043844 0.043844 0.043844
  spline S98 degree 3 poles (-271.1987, 103.651) (-271.0998, 103.6444) (-270.9107, 103.6319) (-270.7644, 103.5123) (-270.6946, 103.4552) knots 0 0 0 0 0.028913 0.055291 0.055291 0.055291 0.055291
  spline S99 degree 3 poles (-270.6946, 103.4552) (-270.6404, 103.3795) (-270.5232, 103.2161) (-270.5136, 103.0144) (-270.5084, 102.9061) knots 0 0 0 0 0.027351 0.059089 0.059089 0.059089 0.059089
  spline S100 degree 3 poles (-270.5084, 102.9061) (-270.5135, 102.7942) (-270.523, 102.5864) (-270.6418, 102.4168) (-270.6967, 102.3386) knots 0 0 0 0 0.032809 0.060899 0.060899 0.060899 0.060899
  spline S101 degree 3 poles (-270.6967, 102.3386) (-270.7652, 102.2797) (-270.9056, 102.1591) (-271.0905, 102.1442) (-271.1851, 102.1367) knots 0 0 0 0 0.026399 0.05408 0.05408 0.05408 0.05408
  spline S102 degree 3 poles (-270.7621, 102.9566) (-270.7692, 103.0293) (-270.7823, 103.1635) (-270.8611, 103.2724) (-270.8972, 103.3222) knots 0 0 0 0 0.021465 0.039604 0.039604 0.039604 0.039604
  spline S103 degree 3 poles (-270.8972, 103.3222) (-270.9405, 103.3592) (-271.0278, 103.4339) (-271.1423, 103.444) (-271.2001, 103.4491) knots 0 0 0 0 0.016633 0.033577 0.033577 0.033577 0.033577
  spline S104 degree 3 poles (-271.2001, 103.4491) (-271.2429, 103.4465) (-271.3256, 103.4416) (-271.3964, 103.3988) (-271.4306, 103.3781) knots 0 0 0 0 0.012642 0.024448 0.024448 0.024448 0.024448
  spline S105 degree 3 poles (-272.4606, 51.4561) (-272.4904, 51.4358) (-272.5491, 51.3959) (-272.5817, 51.3329) (-272.5977, 51.3019) knots 0 0 0 0 0.010635 0.020922 0.020922 0.020922 0.020922
  spline S106 degree 3 poles (-272.5977, 51.3019) (-272.6094, 51.2623) (-272.6366, 51.1701) (-272.6375, 51.0738) (-272.638, 51.0188) knots 0 0 0 0 0.012329 0.028714 0.028714 0.028714 0.028714
  line L93 (-272.638, 51.0188) -> (-272.638, 50.2426)
  line L94 (-272.638, 50.2426) -> (-272.8835, 50.2426)
  spline S107 degree 3 poles (-273.7894, 51.7242) (-273.7043, 51.7218) (-273.5507, 51.7174) (-273.4181, 51.641) (-273.359, 51.6068) knots 0 0 0 0 0.025053 0.045234 0.045234 0.045234 0.045234
  spline S108 degree 3 poles (-273.359, 51.6068) (-273.3138, 51.561) (-273.2177, 51.4635) (-273.1865, 51.3298) (-273.17, 51.259) knots 0 0 0 0 0.01895 0.040278 0.040278 0.040278 0.040278
  line L95 (-273.17, 51.259) -> (-273.4129, 51.2208)
  spline S109 degree 3 poles (-272.7158, 103.6155) (-272.6831, 103.6219) (-272.6218, 103.6338) (-272.5594, 103.6362) (-272.5302, 103.6373) knots 0 0 0 0 0.009958 0.018706 0.018706 0.018706 0.018706
  spline S110 degree 3 poles (-272.5302, 103.6373) (-272.4901, 103.6366) (-272.4181, 103.6352) (-272.352, 103.6073) (-272.3229, 103.595) knots 0 0 0 0 0.011916 0.021334 0.021334 0.021334 0.021334
  spline S111 degree 3 poles (-272.3229, 103.595) (-272.3003, 103.5802) (-272.2566, 103.5516) (-272.2314, 103.5059) (-272.2192, 103.4839) knots 0 0 0 0 0.007958 0.015408 0.015408 0.015408 0.015408
  spline S112 degree 3 poles (-272.2192, 103.4839) (-272.2105, 103.4484) (-272.1875, 103.3534) (-272.1885, 103.2553) (-272.1892, 103.194) knots 0 0 0 0 0.010927 0.02924 0.02924 0.02924 0.02924
  spline S113 degree 3 poles (-272.4334, 103.2076) (-272.433, 103.2365) (-272.4324, 103.2821) (-272.4426, 103.3265) (-272.4463, 103.3427) knots 0 0 0 0 0.008635 0.013608 0.013608 0.013608 0.013608
  spline S114 degree 3 poles (-272.4886, 103.3904) (-272.5003, 103.3956) (-272.527, 103.4073) (-272.5562, 103.4078) (-272.5725, 103.4081) knots 0 0 0 0 0.003804 0.008651 0.008651 0.008651 0.008651
  spline S115 degree 3 poles (-273.9838, 50.4745) (-273.953, 50.4562) (-273.885, 50.4159) (-273.8056, 50.4132) (-273.7621, 50.4118) knots 0 0 0 0 0.01057 0.023371 0.023371 0.023371 0.023371
  spline S116 degree 3 poles (-273.7621, 50.4118) (-273.7127, 50.4121) (-273.6276, 50.4128) (-273.5522, 50.4515) (-273.5206, 50.4677) knots 0 0 0 0 0.014563 0.025087 0.025087 0.025087 0.025087
  spline S117 degree 3 poles (-273.5206, 50.4677) (-273.4996, 50.4863) (-273.4597, 50.5216) (-273.452, 50.574) (-273.4483, 50.5987) knots 0 0 0 0 0.00814 0.015395 0.015395 0.015395 0.015395
  spline S118 degree 3 poles (-273.4483, 50.5987) (-273.4496, 50.6142) (-273.4522, 50.6454) (-273.4696, 50.6715) (-273.4784, 50.6846) knots 0 0 0 0 0.004598 0.009239 0.009239 0.009239 0.009239
  spline S119 degree 3 poles (-273.4784, 50.6846) (-273.4906, 50.6975) (-273.5173, 50.7258) (-273.5531, 50.7415) (-273.5725, 50.7501) knots 0 0 0 0 0.005284 0.01157 0.01157 0.01157 0.01157
  spline S120 degree 3 poles (-273.5725, 50.7501) (-273.5967, 50.7577) (-273.6685, 50.7803) (-273.7412, 50.7999) (-273.7894, 50.8128) knots 0 0 0 0 0.007605 0.022583 0.022583 0.022583 0.022583
  spline S121 degree 3 poles (-273.7894, 50.8128) (-273.8636, 50.8325) (-273.9865, 50.8652) (-274.1057, 50.9093) (-274.153, 50.9268) knots 0 0 0 0 0.023005 0.038118 0.038118 0.038118 0.038118
  spline S122 degree 3 poles (-274.153, 50.9268) (-274.1852, 50.9429) (-274.2483, 50.9744) (-274.2929, 51.029) (-274.3146, 51.0557) knots 0 0 0 0 0.010681 0.020888 0.020888 0.020888 0.020888
  spline S123 degree 3 poles (-274.3146, 51.0557) (-274.3317, 51.0866) (-274.3678, 51.1518) (-274.3714, 51.2265) (-274.3733, 51.2658) knots 0 0 0 0 0.010453 0.022074 0.022074 0.022074 0.022074
  spline S124 degree 3 poles (-274.3733, 51.2658) (-274.3701, 51.3064) (-274.3637, 51.3888) (-274.3226, 51.4606) (-274.3017, 51.497) knots 0 0 0 0 0.012054 0.024479 0.024479 0.024479 0.024479
  spline S125 degree 3 poles (-274.3017, 51.497) (-274.2745, 51.5314) (-274.2181, 51.6027) (-274.1369, 51.6436) (-274.095, 51.6648) knots 0 0 0 0 0.013001 0.026908 0.026908 0.026908 0.026908
  spline S126 degree 3 poles (-274.095, 51.6648) (-274.0475, 51.6821) (-273.9489, 51.7181) (-273.8439, 51.7221) (-273.7894, 51.7242) knots 0 0 0 0 0.015065 0.0313 0.0313 0.0313 0.0313
  spline S127 degree 3 poles (-268.9524, 51.4636) (-268.9641, 51.4687) (-268.9908, 51.4805) (-269.02, 51.481) (-269.0363, 51.4813) knots 0 0 0 0 0.003804 0.008651 0.008651 0.008651 0.008651
  spline S128 degree 3 poles (-269.0363, 51.4813) (-269.0522, 51.4808) (-269.0882, 51.4795) (-269.124, 51.4745) (-269.1441, 51.4718) knots 0 0 0 0 0.004747 0.010826 0.010826 0.010826 0.010826
  line L96 (-269.1441, 51.4718) -> (-269.1796, 51.6887)
  spline S129 degree 3 poles (-267.256, 102.1639) (-267.2506, 102.2317) (-267.2401, 102.365) (-267.1584, 102.4707) (-267.1182, 102.5227) knots 0 0 0 0 0.019911 0.039185 0.039185 0.039185 0.039185
  spline S130 degree 3 poles (-267.1182, 102.5227) (-267.062, 102.5674) (-266.9372, 102.6667) (-266.7793, 102.6935) (-266.6926, 102.7083) knots 0 0 0 0 0.021209 0.047103 0.047103 0.047103 0.047103
  spline S131 degree 3 poles (-266.6926, 102.7083) (-266.7241, 102.7239) (-266.7806, 102.7518) (-266.8302, 102.7907) (-266.8522, 102.8079) knots 0 0 0 0 0.010515 0.018858 0.018858 0.018858 0.018858
  spline S132 degree 3 poles (-266.8522, 102.8079) (-266.8911, 102.8467) (-266.9728, 102.9283) (-267.0378, 103.0239) (-267.0718, 103.0739) knots 0 0 0 0 0.016455 0.034567 0.034567 0.034567 0.034567
  line L97 (-267.0718, 103.0739) -> (-267.4197, 103.6182)
  line L98 (-267.4197, 103.6182) -> (-267.0868, 103.6182)
  line L99 (-267.0868, 103.6182) -> (-266.8222, 103.2021)
  line L100 (-266.2287, 102.7301) -> (-265.9218, 102.7301)
  line L101 (-265.9218, 102.7301) -> (-265.9218, 103.6182)
  line L102 (-269.1441, 50.4336) -> (-268.8972, 50.4336)
  line L103 (-268.8972, 50.4336) -> (-268.8972, 51.2808)
  spline S133 degree 3 poles (-268.8972, 51.2808) (-268.8968, 51.3097) (-268.8962, 51.3553) (-268.9064, 51.3996) (-268.9101, 51.4158) knots 0 0 0 0 0.008635 0.013608 0.013608 0.013608 0.013608
  spline S134 degree 3 poles (-268.9101, 51.4158) (-268.9152, 51.4254) (-268.9255, 51.4447) (-268.9434, 51.4572) (-268.9524, 51.4636) knots 0 0 0 0 0.003189 0.00646 0.00646 0.00646 0.00646
  spline S135 degree 3 poles (-283.8822, 51.768) (-283.925, 51.7654) (-284.0078, 51.7606) (-284.0786, 51.7177) (-284.1128, 51.697) knots 0 0 0 0 0.012642 0.024448 0.024448 0.024448 0.024448
  spline S136 degree 3 poles (-284.1128, 51.697) (-284.1436, 51.6679) (-284.2112, 51.6042) (-284.2455, 51.5176) (-284.2642, 51.4706) knots 0 0 0 0 0.012573 0.027537 0.027537 0.027537 0.027537
  line L104 (-284.2642, 51.4706) -> (-284.518, 51.5019)
  spline S137 degree 3 poles (-284.518, 51.5019) (-284.4947, 51.5712) (-284.4495, 51.7052) (-284.3458, 51.8009) (-284.2956, 51.8471) knots 0 0 0 0 0.021523 0.041652 0.041652 0.041652 0.041652
  spline S138 degree 3 poles (-284.2956, 51.8471) (-284.2355, 51.8829) (-284.108, 51.9588) (-283.9595, 51.9661) (-283.8809, 51.9699) knots 0 0 0 0 0.020652 0.043844 0.043844 0.043844 0.043844
  spline S139 degree 3 poles (-283.8809, 51.9699) (-283.782, 51.9633) (-283.5929, 51.9508) (-283.4466, 51.8312) (-283.3768, 51.7741) knots 0 0 0 0 0.028913 0.055291 0.055291 0.055291 0.055291
  spline S140 degree 3 poles (-283.3768, 51.7741) (-283.3225, 51.6985) (-283.2054, 51.535) (-283.1957, 51.3333) (-283.1906, 51.225) knots 0 0 0 0 0.027351 0.059089 0.059089 0.059089 0.059089